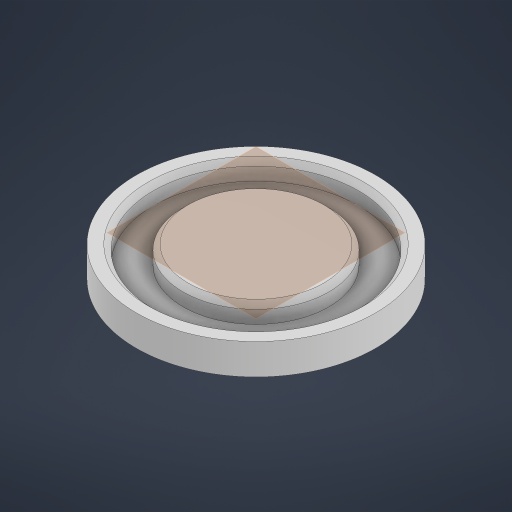
# Autodesk Inventor part: Spinner_Base
Saved by Autodesk Inventor 2023.4 (Build 274418000, 418)
## iProperties
Created: 2025-03-29
Part Number: Spinner_Base
Material: Generic
Document SubType Name: Modeling
Designer: Simon
Density: 1 g/cm^3
Appearance: Default
Author: Simon
Autodesk Inventor part; units mm, degrees
ref_plane "YZ Plane" through (0, 0, 0) normal (1, 0, 0) x (0, 1, 0)
ref_plane "XZ Plane" through (0, 0, 0) normal (0, 1, 0) x (-1, 0, 0)
ref_plane "XY Plane" through (0, 0, 0) normal (0, 0, 1) x (1, 0, 0)
sketch "Sketch1" plane through (0, 0, 0) normal (1, 0, 0) x (0, 1, 0)
  line L0 (1.91, 21.4) -> (-1.91, 21.4)
  line L1 (-1.91, 21.4) -> (-1.91, 30.1)
  line L2 (-1.91, 30.1) -> (1.91, 30.1)
  line L3 (1.91, 21.4) -> (1.91, 0)
  line L4 (1.91, 30.1) -> (1.91, 35.1)
  line L5 (1.91, 35.1) -> (-5.59, 35.1)
  line L6 (-5.59, 35.1) -> (-5.59, 0)
  line L7 (-5.59, 0) -> (1.91, 0)
  point P0 (0, 0)
  dimension "d4" = 5
  dimension "d5" = 7.5
  constraints: 16 end point, 2 perpendicular, 2 vertical, 1 horizontal, 1 parallel
  measures "d4" distance of L2.end L4.end
  measures "d5" distance of L4.end L5.end
revolve "Revolution1" add sketch "Sketch1" angle 360 about axis through (0, -5.59, 0) along (0, 1, 0)
chamfer "Chamfer1" distance 1.5 angle 45 2 edges at (0, 1.91, -30.1) (0, 1.91, -21.4)
move faces "Move1" translate (0, 1.5, 0) faces at (6.585, 1.91, -0.7996) (-3.3526, 0.91, 20.6294) (-2.5025, 1.41, 30.9992) (3.8791, 1.91, -32.3815)
ref_plane "Work Plane1" through (0, 6.29, 0) normal (0, 1, 0) x (1, 0, 0)
body "Solid1"
